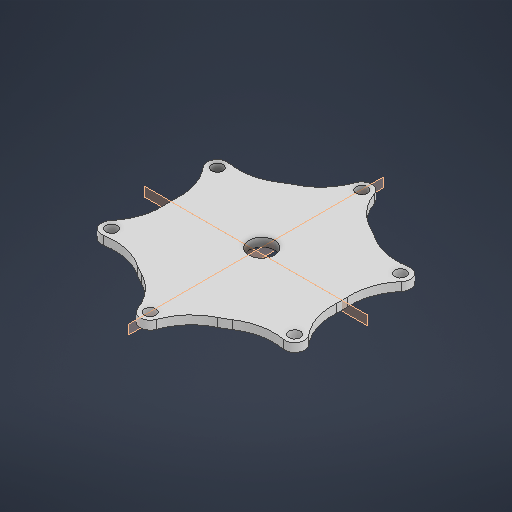
# Autodesk Inventor part: carcaza motor
Saved by Autodesk Inventor 2025.3 (Build 293356000, 356)
## iProperties
Created: 2025-10-02
Part Number: carcaza motor
Material: Generic
Document SubType Name: Modeling
Designer: sophi
Density: 1 g/cm^3
Appearance: Default
Author: sophi
Autodesk Inventor part; units mm, degrees
ref_plane "XZ Plane" through (0, 0, 0) normal (0, 1, 0) x (-1, 0, 0)
sketch "Sketch1" plane through (0, 0, 0) normal (0, 1, 0) x (-1, 0, 0)
  circle A0 centre (0, 0) radius 30
  circle A1 centre (0, 0) radius 27.5
  circle A2 centre (0, -37) radius 3.5
  arc A3 (13.2962, -26.8926) -> (3.3005, -38.1648) centre (22.1604, -44.8209) ccw
  line L0 (0, -39.6745) -> (0, -15.9391) construction
  arc A4 (-3.3005, -38.1648) -> (-13.2962, -26.8926) centre (-22.1604, -44.8209) ccw
  line L1 (47.8103, 0) -> (-62.0389, 0) construction
  circle A5 centre (0, -37) radius 2
  circle A6 centre (32.0429, -18.5) radius 3.5
  circle A7 centre (32.0429, -18.5) radius 2
  arc A8 (31.4015, -21.9407) -> (16.6415, -24.9612) centre (27.7359, -41.6019) ccw
  arc A9 (29.9378, -1.9314) -> (34.7019, -16.2241) centre (49.8963, -3.219) ccw
  circle A10 centre (32.0429, 18.5) radius 3.5
  circle A11 centre (32.0429, 18.5) radius 2
  arc A12 (34.7019, 16.2241) -> (29.9378, 1.9314) centre (49.8963, 3.219) ccw
  arc A13 (16.6415, 24.9612) -> (31.4015, 21.9407) centre (27.7359, 41.6019) ccw
  circle A14 centre (0, 37) radius 3.5
  circle A15 centre (0, 37) radius 2
  arc A16 (3.3005, 38.1648) -> (13.2962, 26.8926) centre (22.1604, 44.8209) ccw
  arc A17 (-13.2962, 26.8926) -> (-3.3005, 38.1648) centre (-22.1604, 44.8209) ccw
  circle A18 centre (-32.0429, 18.5) radius 3.5
  circle A19 centre (-32.0429, 18.5) radius 2
  arc A20 (-31.4015, 21.9407) -> (-16.6415, 24.9612) centre (-27.7359, 41.6019) ccw
  arc A21 (-29.9378, 1.9314) -> (-34.7019, 16.2241) centre (-49.8963, 3.219) ccw
  circle A22 centre (-32.0429, -18.5) radius 3.5
  circle A23 centre (-32.0429, -18.5) radius 2
  arc A24 (-34.7019, -16.2241) -> (-29.9378, -1.9314) centre (-49.8963, -3.219) ccw
  arc A25 (-16.6415, -24.9612) -> (-31.4015, -21.9407) centre (-27.7359, -41.6019) ccw
  point P0 (29.9378, 1.9314)
  point P1 (34.7019, 16.2241)
  point P2 (16.6415, 24.9612)
  point P3 (13.2962, 26.8926)
  point P4 (3.3005, 38.1648)
  point P5 (-13.2962, 26.8926)
  point P6 (-29.9378, 1.9314)
  point P7 (-29.9378, -1.9314)
  point P8 (-16.6415, -24.9612)
  point P9 (-13.2962, -26.8926)
  point P10 (-3.3005, -38.1648)
  point P11 (16.6415, -24.9612)
  point P12 (31.4015, -21.9407)
  point P13 (29.9378, -1.9314)
  dimension "d16" = 60
  dimension "d18" = 7
  dimension "d17" = 55
  dimension "d19" = 37
  dimension "d21" = 20
  dimension "d22" = 4
  dimension "d25" = 360
  constraints: 24 point on circle, 19 centre point, 8 coincident, 4 end point, 3 symmetric about line, 2 point on line, 1 horizontal, 1 vertical, 1 vertical alignment, 97 other
  measures "d17" diameter of A1
  measures "d19" distance of point (0, 0) point (0, -37)
  measures "d21" radius of A3
  measures "d22" diameter of A5
extrude "Extrusion5" add sketch "Sketch1" along normal blind 3
extrude "Extrusion6" add sketch "Sketch1" along normal blind 3 contours A1
sketch "Sketch10" plane through (0, 3, 0) normal (0, 1, 0) x (1, 0, 0)
  circle A0 centre (0, 2) radius 4.5
  circle A1 centre (0, 2) radius 22.5
  point P0 (0, 0)
  dimension "d58" = 9
  dimension "d59" = 45
  dimension "d60" = 2
  constraints: 2 centre point, 1 concentric, 1 vertical alignment
  measures "d58" diameter of A0
  measures "d59" diameter of A1
  measures "d60" distance of A0.centre point (0, 0)
extrude "Extrusion12" cut sketch "Sketch10" against normal blind 20.25 contours A0
body "Solid2"
